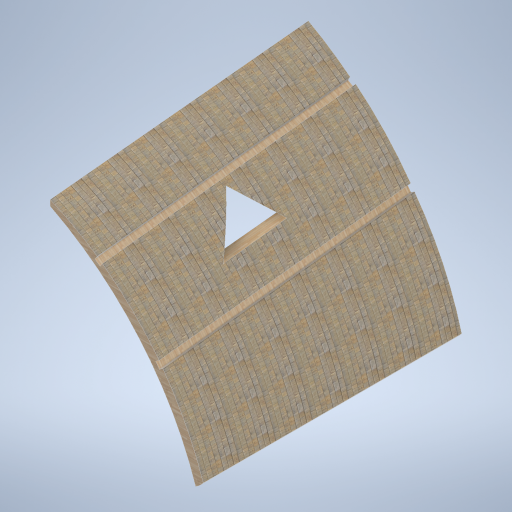
# Autodesk Inventor part: panel_block_02
Saved by Autodesk Inventor 2024.2 (Build 282272000, 272)
## iProperties
Created: 2024-05-21
Part Number: panel_block_02
Material: Wood (Maple)
Document SubType Name: Modeling
Designer: LOSTER_1
Density: 0.67 g/cm^3
Appearance: Natural Maple - Glossy Dark Tint
Author: LOSTER_1
Autodesk Inventor part; units mm, degrees
ref_plane "XZ Plane" through (0, 0, 0) normal (0, 1, 0) x (-1, 0, 0)
sketch "Sketch1" plane through (0, 0, 0) normal (0, 0, 1) x (1, 0, 0)
  line L0 (2948.6488, 634.5525) -> (2841.4489, 559.4904)
  line L1 (2841.4489, 559.4904) -> (2956.2003, 395.6085)
  line L2 (2956.2003, 395.6085) -> (3063.4001, 470.6706)
  line L3 (1051.1773, 2444.1167) -> (976.8907, 2338.0244)
  line L4 (976.8907, 2338.0244) -> (1140.7211, 2223.3091)
  line L5 (1140.7211, 2223.3091) -> (1215.0077, 2329.4014)
  line L6 (-383.8501, 3232.1868) -> (-383.8501, 3052.6308)
  arc A0 (4065.9398, -2152.4924) -> (-383.8501, 3052.6308) centre (-4485.4868, -4958.3977) ccw
  arc A1 (1051.1773, 2444.1167) -> (-383.8501, 3232.1868) centre (-3980.604, -5017.8654) ccw
  arc A2 (2948.6488, 634.5525) -> (1215.0077, 2329.4014) centre (-4152.392, -4894.9339) ccw
  arc A3 (4300.883, -1939.8955) -> (3063.4001, 470.6706) centre (-4233.2291, -4798.0297) ccw
  arc A4 (4065.9398, -2152.4924) -> (4300.883, -1939.8955) centre (3657.2708, -1464.7499) ccw
  point P0 (0, 0)
  point P1 (4065.924, -2152.4924)
  point P2 (4065.924, -2152.4924)
  dimension "d8" = 9000
  dimension "d9" = 9000
  dimension "d10" = 9000
  dimension "d11" = 9000
  dimension "d12" = 800
  constraints: 14 end point, 10 point on circle, 5 centre point, 4 perpendicular, 1 coincident, 1 vertical
  measures "d8" radius of A0
  measures "d9" radius of A1
  measures "d10" radius of A2
  measures "d11" radius of A3
  measures "d12" radius of A4
ref_plane "Work Plane2" through (0, 0, -7900) normal (0, 0, 1) x (1, 0, 0)
ref_plane "Work Plane1" through (0, 0, 0) normal (0, 0, 1) x (1, 0, 0)
sketch "Sketch2" plane through (0, 0, -7900) normal (0, 0, 1) x (1, 0, 0)
  arc A0 (895.257, 3171.2695) -> (-383.8658, 4018.7524) centre (-4697.1096, -3880.3569) ccw projected
  line L0 (-383.8658, 4018.7524) -> (-383.8658, 3839.1061) projected
  arc A1 (4065.924, -2152.4924) -> (-383.8658, 3839.1061) centre (-4733.9746, -4039.7614) ccw projected
  line L1 (895.257, 3171.2695) -> (830.4728, 3059.0601) projected
  line L2 (830.4728, 3059.0601) -> (1003.6891, 2959.0536) projected
  line L3 (1068.4733, 3071.2631) -> (1003.6891, 2959.0536) projected
  arc A2 (2750.1419, 1279.62) -> (1068.4733, 3071.2631) centre (-4591.4319, -3926.2703) ccw projected
  line L4 (2750.1419, 1279.62) -> (2643.8882, 1205.2246) projected
  line L5 (2643.8882, 1205.2246) -> (2759.146, 1041.7698) projected
  line L6 (2865.5448, 1116.2711) -> (2759.146, 1041.7698) projected
  arc A3 (4310.9102, -1926.005) -> (2865.5448, 1116.2711) centre (-4397.3898, -4198.7812) ccw projected
  arc A4 (4065.924, -2152.4924) -> (4310.9102, -1926.005) centre (3657.2831, -1464.7333) ccw
  point P0 (0, 0)
  dimension "d7" = 800
  constraints: 2 point on circle, 1 centre point
  measures "d7" radius of A4
loft "Loft1" add profiles "Sketch1", "Sketch2"
ref_plane "Work Plane3" through (2500, 0, 0) normal (1, 0, 0) x (0, 1, 0)
sketch "Sketch3" plane through (2500, 0, 0) normal (1, 0, 0) x (0, 1, 0)
  line L0 (2569.5835, -3718.0946) -> (1551.2045, -2616.5476)
  line L1 (1551.2045, -2616.5476) -> (1738.7871, -4630.7013)
  line L2 (1738.7871, -4630.7013) -> (2569.5835, -3718.0946)
  point P0 (0, 0)
  constraints: 6 end point
extrude "Extrusion1" cut sketch "Sketch3" against normal through all
body "Solid1"
